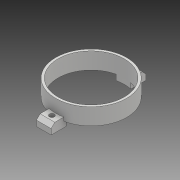
# Autodesk Inventor part: conectcover
Saved by Autodesk Inventor 2018 (Build 220112000, 112)
## iProperties
Created: 2019-02-27
Part Number: conectcover
Material: 一般
Document SubType Name: Modeling
Designer: ku_sk
Density: 1 g/cm^3
Appearance: 既定
Author: ku_sk
Autodesk Inventor part; units mm, degrees
ref_plane "YZ Plane" through (0, 0, 0) normal (1, 0, 0) x (0, 1, 0)
ref_plane "XZ Plane" through (0, 0, 0) normal (0, 1, 0) x (-1, 0, 0)
ref_plane "XY Plane" through (0, 0, 0) normal (0, 0, 1) x (1, 0, 0)
sketch "スケッチ1" plane through (0, 0, 0) normal (0, 0, 1) x (1, 0, 0)
  line L0 (-4, 25.75) -> (4, 25.75)
  line L1 (4, 25.75) -> (4, 17.5499)
  line L2 (-4, 17.5499) -> (-4, 25.75)
  line L3 (4, -17.5499) -> (4, -25.75)
  line L4 (4, -25.75) -> (-4, -25.75)
  line L5 (-4, -25.75) -> (-4, -17.5499)
  line L6 (0, -36.05) -> (0, 36.05) projected
  arc A0 (4, 17.5499) -> (-4, 17.5499) centre (0, 0) ccw
  arc A1 (-4, -17.5499) -> (4, -17.5499) centre (0, 0) ccw
  point P0 (0, 18)
  dimension "d1" = 18
  dimension "d2" = 18
  dimension "d3" = 51.5
  dimension "d4" = 25.75
  dimension "d5" = 8
  constraints: 12 end point, 5 point on circle, 3 point on line, 2 centre point, 2 coincident, 2 parallel, 1 collinear, 1 horizontal, 1 perpendicular
  measures "d1" radius of A1
  measures "d2" radius of A0
  measures "d3" distance between parallel lines of L4 L0
  measures "d4" distance from line of point (0, 0) L0
  measures "d5" distance of L0.start L0.end
extrude "押し出し1" add sketch "スケッチ1" along normal blind 5
chamfer "面取り1" distance 2 angle 45 2 edges at (0, 25.75, 5) (0, -25.75, 5)
sketch "スケッチ2" plane through (0, 0, 5) normal (0, 0, 1) x (1, 0, 0)
  line L0 (4, 25.75) -> (4, 17.5499) projected
  circle A0 centre (0, 0) radius 18
  circle A1 centre (0, 0) radius 19.25
  dimension "d15" = 38.5
  constraints: 1 centre point, 1 coincident, 3 other
  measures "d15" diameter of A1
extrude "押し出し2" add sketch "スケッチ2" along normal blind 7 and the other way blind 2
sketch "スケッチ3" plane through (0, 0, 3) normal (0, 0, -1) x (-1, 0, 0)
  line L0 (18.6548, 4.75) -> (20.5, 4.75)
  line L1 (20.5, 4.75) -> (20.5, -4.75)
  line L2 (20.5, -4.75) -> (18.6548, -4.75)
  arc A0 (4, -18.8298) -> (4, 18.8298) centre (0, 0) ccw projected
  line L3 (28.45, 0) -> (-27.2, 0) projected
  arc A1 (4, -17.5499) -> (4, 17.5499) centre (0, 0) ccw projected
  point P0 (20.5, 0)
  point P1 (18, 0)
  dimension "d16" = 9.5
  dimension "d17" = 2.5
  constraints: 6 end point, 3 point on circle, 2 perpendicular, 2 point on line, 1 horizontal, 1 midpoint
  measures "d16" distance between parallel lines of L2 L0
  measures "d17" distance from line of L1 point (18, 0)
extrude "押し出し3" add sketch "スケッチ3" against normal blind 1.8
chamfer "面取り2" distance 1.84 angle 45 2 edges at (-20.5, 4.75, 3.9) (-20.5, -4.75, 3.9)
sketch "スケッチ4" plane through (0, 0, 5) normal (0, 0, 1) x (1, 0, 0)
  circle A0 centre (0, 21.35) radius 1.35
  circle A1 centre (0, -21.35) radius 1.35
  line L0 (0, 20) -> (0, -20)
  point P0 (0, 0)
  point P1 (0, 0)
  dimension "d23" = 2.7
  dimension "d24" = 2.7
  dimension "d25" = 40
  constraints: 2 end point, 2 point on line, 2 vertical alignment, 1 coincident, 1 midpoint, 1 vertical, 4 other
  measures "d25" distance of L0.start L0.end
extrude "押し出し4" cut sketch "スケッチ4" against normal up to surface (5 mm away)
equation "\"d4\" = 0.5 * d3"
equation "\"d24\" = d23"
